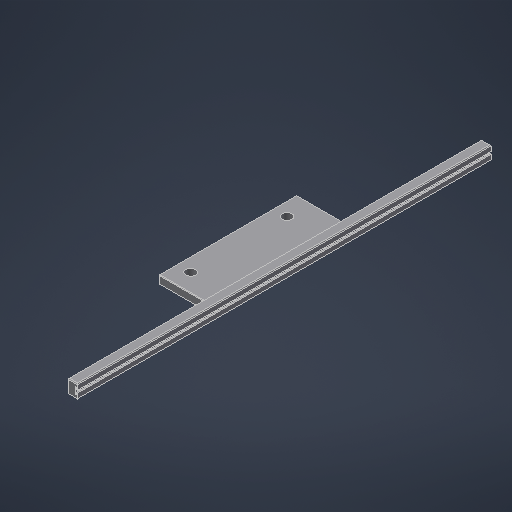
# Autodesk Inventor part: Soporte Boquillas
Saved by Autodesk Inventor 2026 (Build 300175000, 175)
## iProperties
Created: 2025-05-12
Part Number: Soporte Boquillas
Material: Generic
Document SubType Name: Modeling
Designer: feder
Density: 1 g/cm^3
Appearance: Default
Author: feder
Autodesk Inventor part; units mm, degrees
ref_plane "YZ Plane" through (0, 0, 0) normal (1, 0, 0) x (0, 1, 0)
ref_plane "XZ Plane" through (0, 0, 0) normal (0, 1, 0) x (-1, 0, 0)
ref_plane "XY Plane" through (0, 0, 0) normal (0, 0, 1) x (1, 0, 0)
sketch "Sketch1" plane through (0, 0, 0) normal (0, 0, 1) x (1, 0, 0)
  line L0 (-17.5, 25) -> (17.5, 25)
  line L1 (17.5, 25) -> (17.5, -25)
  line L2 (17.5, -25) -> (-17.5, -25)
  line L3 (-17.5, -25) -> (-17.5, 25)
  line L4 (17.5, 4.5) -> (12.5, 4.5)
  line L5 (12.5, 4.5) -> (12.5, -4.5)
  line L6 (12.5, -4.5) -> (17.5, -4.5)
  line L7 (17.5, -4.5) -> (17.5, 4.5)
  line L8 (12.5, 12.5) -> (9.5, 12.5)
  line L9 (9.5, 12.5) -> (9.5, -12.5)
  line L10 (9.5, -12.5) -> (12.5, -12.5)
  line L11 (12.5, -12.5) -> (12.5, 12.5)
  point P0 (0, 0)
  point P1 (0, 25)
  point P2 (-17.5, 0)
  point P3 (12.5, 0)
  point P4 (9.5, 0)
  dimension "d0" = 35
  dimension "d1" = 50
  dimension "d7" = 5
  dimension "d8" = 9
  dimension "d9" = 3
  dimension "d10" = 25
  constraints: 24 end point, 6 parallel, 4 midpoint, 3 horizontal alignment, 3 perpendicular, 2 horizontal, 2 point on line, 1 vertical, 1 vertical alignment
  measures "d0" distance of L0.start L0.end
  measures "d1" distance of L2.end L0.start
  measures "d7" distance of L6.end L5.end
  measures "d8" distance of L4.end L5.end
  measures "d9" distance of L10.end L9.end
  measures "d10" distance of L8.end L9.end
extrude "Extrusion1" add sketch "Sketch1" along normal blind 1500 contours L0 L1 L4 L11 L8 L9 L10 L6 L2 L3
fillet "Fillet2" radius 3 10 edges at (17.5, 25, 750) (-17.5, 25, 750) (0, 25, 1500) (-17.5, 0, 1500) (0, -25, 1500) (-17.5, -25, 750) (17.5, -25, 750) (-17.5, 0, 0) (0, 25, 0) (0, -25, 0)
sketch "Sketch3" plane through (-17.5, -22, 3) normal (-1, 0, 0) x (0, 0, 1)
  line L0 (497, 37) -> (997, 37)
  line L1 (997, 37) -> (997, 7)
  line L2 (997, 7) -> (497, 7)
  line L3 (497, 7) -> (497, 37)
  point P0 (-3, 22)
  point P1 (497, 22)
  point P2 (747, 37)
  dimension "d12" = 500
  dimension "d13" = 30
  dimension "d14" = 750
  constraints: 8 end point, 2 midpoint, 2 parallel, 1 horizontal, 1 horizontal alignment, 1 perpendicular
  measures "d12" distance of L1.end L2.end
  measures "d13" distance of L0.end L1.end
  measures "d14" horizontal distance of point (747, 37) point (-3, 22)
extrude "Extrusion2" add sketch "Sketch3" along normal blind 170
fillet "Fillet3" radius 2 8 edges at (-102.5, -15, 500) (-102.5, 15, 500) (-102.5, 15, 1000) (-102.5, -15, 1000) (-187.5, 15, 750) (-187.5, -15, 750) (-187.5, 0, 500) (-187.5, 0, 1000)
sketch "Sketch4" plane through (-17.5, 15, 998) normal (0, 1, 0) x (1, 0, 0)
  circle A0 centre (-120, 63.5059) radius 17.5
  circle A1 centre (-120, 413.5059) radius 17.5
  line L0 (0, 0) -> (-168, 0) projected
  line L1 (0, 496) -> (0, 0) projected
  point P0 (17.5, 998)
  point P1 (-84, 0)
  point P2 (-84, 0)
  dimension "d18" = 35
  dimension "d19" = 35
  dimension "d20" = 350
  dimension "d21" = 73
  dimension "d24" = 120
  constraints: 2 centre point, 2 midpoint, 1 vertical alignment
  measures "d18" diameter of A0
  measures "d19" diameter of A1
  measures "d20" distance of A1.centre A0.centre
  measures "d21" distance of point (-84, 0) A0.centre
  measures "d24" distance from line of L1 A0.centre
extrude "Extrusion3" cut sketch "Sketch4" against normal blind 150
body "Solid1"
